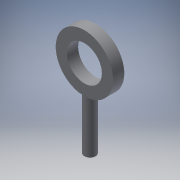
# Autodesk Inventor part: EyeBolt
Saved by Autodesk Inventor 2017 (Build 210142000, 142)
## iProperties
Created: 2017-03-13
Part Number: EyeBolt
Material: Generic
Document SubType Name: Modeling
Designer: Joseph
Density: 1 g/cm^3
Appearance: Default
Author: Joseph
Autodesk Inventor part; units mm, degrees
ref_plane "YZ Plane" through (0, 0, 0) normal (1, 0, 0) x (0, 1, 0)
ref_plane "XZ Plane" through (0, 0, 0) normal (0, 1, 0) x (-1, 0, 0)
ref_plane "XY Plane" through (0, 0, 0) normal (0, 0, 1) x (1, 0, 0)
sketch "Sketch1" plane through (0, 0, 0) normal (0, 1, 0) x (-1, 0, 0)
  circle A0 centre (0, 0) radius 2.032
  dimension "d0" = 4.064
  constraints: 1 centre point, 1 coincident
  measures "d0" diameter of A0
extrude "Extrusion1" add sketch "Sketch1" along normal blind 19.05
sketch "Sketch2" plane through (0, 0, 0) normal (0, 0, 1) x (1, 0, 0)
  circle A0 centre (0, 29.2638) radius 6.35
  line L0 (2.032, 19.05) -> (-2.032, 19.05) projected
  circle A1 centre (0, 29.2638) radius 10.414
  point P0 (0, 0)
  dimension "d3" = 4.064
  dimension "d4" = 12.7
  constraints: 2 centre point, 2 point on circle, 1 coincident
  measures "d3" radial gap between concentric circles of A1 A0
  measures "d4" diameter of A0
extrude "Extrusion2" add sketch "Sketch2" along normal mid plane 4.064 contours L0 A1 picked at (0.2551, 20.3534)
body "Solid1"
